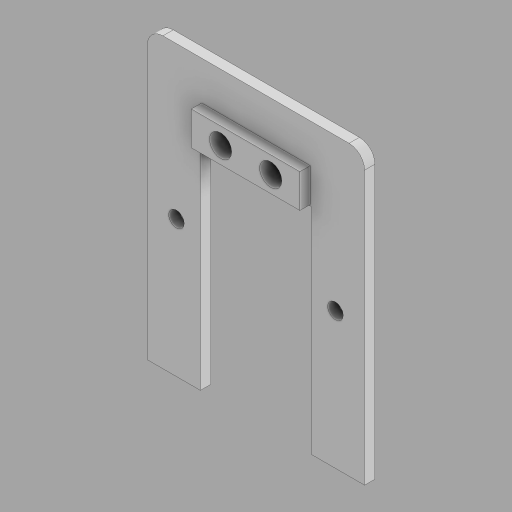
# Autodesk Inventor part: MG995_26_apoio_upgrade
Saved by Autodesk Inventor 2023.2 (Build 272271030, 271C)
## iProperties
Created: 2023-04-15
Part Number: MG995_26_apoio_upgrade
Material: Generic
Document SubType Name: Modeling
Designer: victo
Density: 1 g/cm^3
Appearance: Default
Author: victo
## iProperties of the stored document MG995_26_upgrade_3DPrint.ipt
Created: 2023-06-18
Part Number: MG995_26_upgrade_3DPrint
Material: Generic
Document SubType Name: Modeling
Designer: victo
Density: 1 g/cm^3
Appearance: Default
Author: victo
Autodesk Inventor part; units mm, degrees
ref_plane "YZ Plane" through (0, 0, 0) normal (1, 0, 0) x (0, 1, 0)
ref_plane "XZ Plane" through (0, 0, 0) normal (0, 1, 0) x (-1, 0, 0)
ref_plane "XY Plane" through (0, 0, 0) normal (0, 0, 1) x (1, 0, 0)
sketch "Sketch1" plane through (0, 0, 0) normal (0, 0, 1) x (1, 0, 0)
  line L0 (0, 0) -> (42, 0)
  line L1 (42, 0) -> (42, 70)
  line L2 (42, 70) -> (0, 70)
  line L3 (0, 70) -> (0, 0)
  line L4 (31.75, 14.25) -> (10.25, 14.25)
  line L5 (10.25, 14.25) -> (10.25, 55.75)
  line L6 (10.25, 55.75) -> (31.75, 55.75)
  line L7 (31.75, 55.75) -> (31.75, 14.25)
  line L8 (31.75, 14.25) -> (10.25, 55.75) construction
  line L9 (10.25, 14.25) -> (31.75, 55.75) construction
  line L10 (21, 70) -> (21, 0)
  line L11 (0, 35) -> (42, 35)
  point P0 (21, 35)
  point P1 (10.8, 7)
  point P2 (31.2, 7)
  point P3 (31.2, 0)
  point P4 (10.8, 0)
  point P5 (31.75, 35)
  point P6 (21, 35)
  point P7 (10.25, 35)
  point P8 (21, 14.25)
  point P9 (21, 55.75)
  dimension "d0" = 42
  dimension "d1" = 70
  dimension "d4" = 21.5
  dimension "d5" = 41.5
  constraints: 24 end point, 7 midpoint, 4 parallel, 2 horizontal, 2 perpendicular
  measures "d0" distance of L2.end L1.end
  measures "d1" distance of L1.end L0.end
  measures "d4" distance of L5.end L6.end
  measures "d5" distance of L4.end L5.end
extrude "Extrusion1" add sketch "Sketch1" along normal blind 2
fillet "Fillet3" radius 3 2 edges at (42, 70, 1) (0, 70, 1)
extrude "Extrusion11" cut sketch "Sketch1" along normal blind 6 contours L10 L11 L7 L4 | L4 L5 L11 L10 | L5 L6 L10 L11 | L10 L6 L7 L11
sketch "Sketch14" plane through (0, 0, 2) normal (0, 0, 1) x (1, 0, 0)
  line L0 (31.75, 55.75) -> (10.25, 55.75) projected
  circle A0 centre (16.15, 59.2) radius 2.15
  circle A1 centre (25.85, 59.2) radius 2.15
  line L1 (16.15, 59.2) -> (25.85, 59.2)
  line L2 (10.8, 35) -> (31.2, 35)
  circle A2 centre (16.15, 10.8) radius 2.15
  circle A3 centre (25.85, 10.8) radius 2.15
  line L3 (16.15, 10.8) -> (25.85, 10.8)
  line L4 (0, 0) -> (42, 0) projected
  arc A4 (3, 70) -> (0, 67) centre (3, 67) ccw projected
  line L5 (0, 67) -> (0, 0) projected
  line L6 (42, 0) -> (42, 67) projected
  arc A5 (42, 67) -> (39, 70) centre (39, 67) ccw projected
  line L7 (39, 70) -> (3, 70) projected
  point P0 (21, 59.2)
  dimension "d54" = 4.3
  dimension "d55" = 4.3
  dimension "d56" = 9.7
  constraints: 6 end point, 4 centre point, 2 symmetric about line, 1 horizontal, 1 midpoint, 2 other
  measures "d54" diameter of A0
  measures "d55" diameter of A1
  measures "d56" distance of L1.end L1.start
extrude "Extrusion12" cut sketch "Sketch14" against normal blind 6 contours A0 | A1 | A2 | A3
sketch "Sketch17" plane through (0, 0, 2) normal (0, 0, 1) x (1, 0, 0)
  circle A0 centre (16.15, 10.8) radius 2.15 projected
  circle A1 centre (25.85, 59.2) radius 2.15 projected
  circle A2 centre (25.85, 10.8) radius 2.15 projected
  circle A3 centre (16.15, 59.2) radius 2.15 projected
  line L0 (10.25, 55.75) -> (31.75, 55.75) projected
  line L1 (31.75, 55.75) -> (31.75, 14.25) projected
  line L2 (31.75, 14.25) -> (10.25, 14.25) projected
  line L3 (10.25, 14.25) -> (10.25, 55.75) projected
  circle A4 centre (16.15, 59.2) radius 2.15 projected
  circle A5 centre (25.85, 59.2) radius 2.15 projected
  line L4 (16.15, 61.35) -> (25.85, 61.35)
  line L5 (25.85, 59.2) -> (25.85, 61.35)
  line L6 (14, 59.2) -> (14, 55.75)
  line L7 (28, 59.2) -> (28, 55.75)
  line L8 (10.25, 55.75) -> (10.25, 14.25) projected
  line L9 (10.25, 55.75) -> (10.25, 62.75)
  line L10 (10.25, 62.75) -> (31.75, 62.75)
  line L11 (31.75, 62.75) -> (31.75, 55.75)
  line L12 (0, 0) -> (42, 0) projected
  arc A6 (3, 70) -> (0, 67) centre (3, 67) ccw projected
  line L13 (0, 67) -> (0, 0) projected
  line L14 (42, 0) -> (42, 67) projected
  arc A7 (42, 67) -> (39, 70) centre (39, 67) ccw projected
  line L15 (39, 70) -> (3, 70) projected
  dimension "d67" = 7
  constraints: 14 end point, 5 tangent, 4 perpendicular, 4 point on circle, 2 point on line, 2 vertical
  measures "d67" distance between parallel lines of L0 L10
extrude "Extrusion15" add sketch "Sketch17" along normal blind 2 contours L7 L0 L6 A3 L4 A1 | A1 L4 A3 L6 L0 L9 L10 L11 L7
sketch "Sketch18" plane through (0, 0, 2) normal (0, 0, 1) x (1, 0, 0)
  line L0 (10.25, 14.25) -> (10.25, 55.75) projected
  line L1 (10.25, 62.75) -> (31.75, 62.75) projected
  line L2 (31.75, 55.75) -> (31.75, 14.25) projected
  line L3 (31.75, 14.25) -> (10.25, 14.25) projected
  circle A0 centre (25.85, 10.8) radius 2.15 projected
  circle A1 centre (16.15, 10.8) radius 2.15 projected
  line L4 (10.25, 40.625) -> (5.625, 40.625)
  line L5 (5.625, 40.625) -> (5.625, 69)
  circle A2 centre (5.625, 40.625) radius 1.5
  line L6 (21, 80.706) -> (21, -3.1342)
  circle A3 centre (36.375, 40.625) radius 1.5
  line L7 (0, 0) -> (42, 0) projected
  arc A4 (3, 70) -> (0, 67) centre (3, 67) ccw projected
  line L8 (0, 67) -> (0, 0) projected
  line L9 (42, 0) -> (42, 67) projected
  arc A5 (42, 67) -> (39, 70) centre (39, 67) ccw projected
  line L10 (39, 70) -> (3, 70) projected
  line L11 (10.25, 55.75) -> (10.25, 62.75) projected
  line L12 (31.75, 62.75) -> (31.75, 55.75) projected
  dimension "d70" = 4.625
  dimension "d71" = 28.375
  dimension "d72" = 3
  dimension "d75" = 30.75
  constraints: 6 end point, 2 centre point, 1 coincident, 1 horizontal, 1 point on line, 1 symmetric about line, 1 vertical, 1 other
  measures "d70" distance of L4.start L4.end
  measures "d71" distance of L4.end L5.end
  measures "d72" diameter of A2
  measures "d75" distance of A3.centre L4.end
extrude "Extrusion16" cut sketch "Sketch18" against normal blind 10 contours A2 L5 L4 | L4 L5 A2 | A3
sketch "Sketch22" plane through (0, 0, 2) normal (0, 0, 1) x (1, 0, 0)
  point P0 (0, 0)
sketch "Sketch23" plane through (0, 0, 4) normal (0, 0, 1) x (1, 0, 0)
  line L0 (31.75, 55.75) -> (31.75, 62.75) projected
  line L1 (31.75, 62.75) -> (10.25, 62.75) projected
  line L2 (10.25, 62.75) -> (10.25, 55.75) projected
  line L3 (10.25, 55.75) -> (31.75, 55.75) projected
  circle A0 centre (25.85, 59.2) radius 2.15 projected
  circle A1 centre (16.15, 59.2) radius 2.15 projected
  line L4 (10.5, 56) -> (10.5, 62.5)
  line L5 (10.5, 62.5) -> (31.5, 62.5)
  line L6 (31.5, 62.5) -> (31.5, 56)
  line L7 (31.5, 56) -> (10.5, 56)
  point P0 (0, 0)
  dimension "d88" = 0.25
  constraints: 8 end point, 3 other
  measures "d88" distance between parallel lines of L2 L4
extrude "Extrusion20" cut sketch "Sketch23" against normal blind 2 contours L3 L2 L1 L0
sketch "Sketch24" plane through (0, 0, 2) normal (0, 0, 1) x (1, 0, 0)
  line L0 (10.5, 62.5) -> (10.5, 56) projected
  line L1 (31.5, 62.5) -> (10.5, 62.5) projected
  line L2 (31.5, 56) -> (31.5, 62.5) projected
  line L3 (10.5, 56) -> (31.5, 56) projected
  circle A0 centre (5.625, 40.625) radius 1.5 projected
  circle A1 centre (36.375, 40.625) radius 1.5 projected
  arc A2 (3, 70) -> (0, 67) centre (3, 67) ccw projected
  line L4 (0, 67) -> (0, 0) projected
  line L5 (0, 0) -> (42, 0) projected
  line L6 (42, 0) -> (42, 67) projected
  arc A3 (42, 67) -> (39, 70) centre (39, 67) ccw projected
  line L7 (39, 70) -> (3, 70) projected
  line L8 (31.75, 55.75) -> (10.25, 55.75) projected
  line L9 (31.75, 55.75) -> (31.75, 14.25) projected
  line L10 (31.75, 14.25) -> (10.25, 14.25) projected
  line L11 (10.25, 14.25) -> (10.25, 55.75) projected
  circle A4 centre (25.85, 10.8) radius 2.15 projected
  circle A5 centre (16.15, 10.8) radius 2.15 projected
  line L12 (42, 14.25) -> (0, 14.25)
  line L13 (0, 14.25) -> (0, 0)
  line L14 (0, 0) -> (42, 0)
  line L15 (42, 0) -> (42, 14.25)
  point P0 (31.75, 14.25)
  constraints: 8 end point, 2 parallel, 1 horizontal, 1 perpendicular, 1 point on line
extrude "Extrusion21" cut sketch "Sketch24" against normal blind 10 contours L12 L10 L6 L5 L4
body "Solid1"
